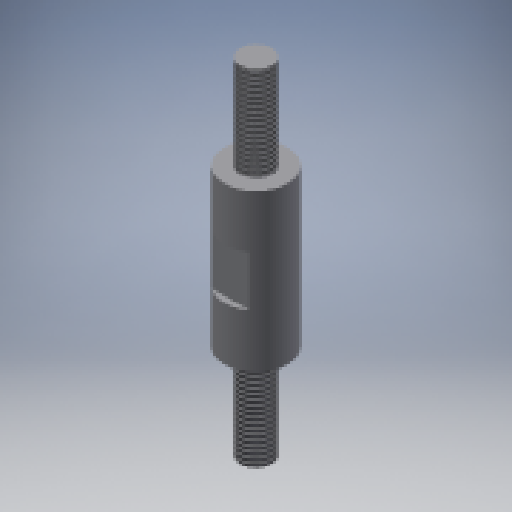
# Autodesk Inventor part: 24_0497_0017
Saved by Autodesk Inventor 2024.3 (Build 283343000, 343)
## iProperties
Created: 2024-06-17
Part Number: 24_0497_0017
Material: Allgemein
Document SubType Name: Modeling
Designer: Vogel
Density: 1 g/cm^3
Appearance: Vorgabe
Author: Vogel
Autodesk Inventor part; units mm, degrees
ref_plane "YZ Plane" through (0, 0, 0) normal (1, 0, 0) x (0, 1, 0)
ref_plane "XZ Plane" through (0, 0, 0) normal (0, 1, 0) x (-1, 0, 0)
ref_plane "XY Plane" through (0, 0, 0) normal (0, 0, 1) x (1, 0, 0)
sketch "Skizze1" plane through (0, 0, 0) normal (0, 0, 1) x (1, 0, 0)
  line L0 (-7, 0) -> (7, 0) projected
  line L1 (0, -7) -> (0, 7) projected
  circle A0 centre (0, 0) radius 5
  dimension "d0" = 10
  constraints: 1 centre point, 1 coincident
  measures "d0" diameter of A0
extrude "Extrusion1" add sketch "Skizze1" along normal mid plane 25
sketch "Skizze2" plane through (0, 0, -12.5) normal (0, 0, -1) x (-1, 0, 0)
  circle A0 centre (0, 0) radius 2.5
  dimension "d3" = 5
  constraints: 1 centre point, 1 coincident
  measures "d3" diameter of A0
extrude "Extrusion2" add sketch "Skizze2" along normal blind 15
sketch "Skizze3" plane through (0, 0, 12.5) normal (0, 0, 1) x (1, 0, 0)
  circle A0 centre (0, 0) radius 2.5
  circle A1 centre (0, 0) radius 2.5 projected
  constraints: 2 concentric, 1 centre point, 1 coincident
extrude "Extrusion3" add sketch "Skizze3" along normal blind 15
thread "Gewinde1" size "M5x0.8" class "6g" standard "ANSI Metric M Profile" full length
sketch "Skizze4" plane through (0, 0, 0) normal (1, 0, 0) x (0, 1, 0)
  line L0 (-7, 0) -> (7, 0) projected
  line L1 (0, -5.6) -> (0, 5.6) projected
  line L2 (-7, 4) -> (-4, 4)
  line L3 (-4, 4) -> (-4, -4)
  line L4 (-4, -4) -> (-7, -4)
  line L5 (-7, -4) -> (-7, 4)
  line L6 (-7, 4) -> (-4, -4) construction
  line L7 (-4, 4) -> (-7, -4) construction
  line L8 (7, 4) -> (4, 4)
  line L9 (4, 4) -> (4, -4)
  line L10 (4, -4) -> (7, -4)
  line L11 (7, -4) -> (7, 4)
  line L12 (7, 4) -> (4, -4) construction
  line L13 (4, 4) -> (7, -4) construction
  point P0 (0, 0)
  point P1 (-5.5, 0)
  point P2 (5.5, 0)
  dimension "d10" = 8
  dimension "d11" = 8
  dimension "d12" = 3
  constraints: 24 end point, 4 midpoint, 4 parallel, 2 equal length, 2 horizontal, 2 perpendicular, 2 point on line, 1 other
  measures "d10" distance between parallel lines of L3 L9
  measures "d11" distance of L4.end L2.start
  measures "d12" distance of L2.start L2.end
extrude "Extrusion4" cut sketch "Skizze4" along normal mid plane 20
